Autodesk Fusion 360 part; units mm, degrees
(part 2 of 4)
sketch "Sketch7" plane through (0, 0, 2.5) normal (0, 0, 1) x (-1, 0, 0)
  line L0 (-32.4248, -53.9298) -> (-46.6248, -53.9298)
  line L1 (-46.6248, -53.9298) -> (-46.6248, -39.7298)
  line L2 (-46.6248, -39.7298) -> (-32.4248, -39.7298)
  line L3 (-32.4248, -39.7298) -> (-32.4248, -53.9298)
  line L4 (5.5752, -42.9298) -> (-8.6248, -42.9298)
  line L5 (-8.6248, -42.9298) -> (-8.6248, -28.7298)
  line L6 (-8.6248, -28.7298) -> (5.5752, -28.7298)
  line L7 (5.5752, -28.7298) -> (5.5752, -42.9298)
  line L8 (-32.4248, -15.9298) -> (-46.6248, -15.9298)
  line L9 (-46.6248, -15.9298) -> (-46.6248, -1.7298)
  line L10 (-46.6248, -1.7298) -> (-32.4248, -1.7298)
  line L11 (-32.4248, -1.7298) -> (-32.4248, -15.9298)
  line L12 (43.5752, 5.0702) -> (29.3752, 5.0702)
  line L13 (29.3752, 5.0702) -> (29.3752, 19.2702)
  line L14 (29.3752, 19.2702) -> (43.5752, 19.2702)
  line L15 (43.5752, 19.2702) -> (43.5752, 5.0702)
  line L16 (69.4872, 20.2441) -> (57.0872, 20.2441)
  line L17 (57.0872, 20.2441) -> (57.0872, 32.3441)
  line L18 (57.0872, 32.3441) -> (69.4872, 32.3441)
  line L19 (69.4872, 32.3441) -> (69.4872, 20.2441)
  line L20 (-13.4248, -57.9298) -> (-27.6248, -57.9298)
  line L21 (-27.6248, -57.9298) -> (-27.6248, -43.7298)
  line L22 (-27.6248, -43.7298) -> (-13.4248, -43.7298)
  line L23 (-13.4248, -43.7298) -> (-13.4248, -57.9298)
  line L24 (-51.4248, -15.9298) -> (-65.6248, -15.9298)
  line L25 (-65.6248, -15.9298) -> (-65.6248, -1.7298)
  line L26 (-65.6248, -1.7298) -> (-51.4248, -1.7298)
  line L27 (-51.4248, -1.7298) -> (-51.4248, -15.9298)
  line L28 (-13.4248, -38.9298) -> (-27.6248, -38.9298)
  line L29 (-27.6248, -38.9298) -> (-27.6248, -24.7298)
  line L30 (-27.6248, -24.7298) -> (-13.4248, -24.7298)
  line L31 (-13.4248, -24.7298) -> (-13.4248, -38.9298)
  line L32 (43.5752, -51.9298) -> (29.3752, -51.9298)
  line L33 (29.3752, -51.9298) -> (29.3752, -37.7298)
  line L34 (29.3752, -37.7298) -> (43.5752, -37.7298)
  line L35 (43.5752, -37.7298) -> (43.5752, -51.9298)
  line L36 (5.5752, -4.9298) -> (-8.6248, -4.9298)
  line L37 (-8.6248, -4.9298) -> (-8.6248, 9.2702)
  line L38 (-8.6248, 9.2702) -> (5.5752, 9.2702)
  line L39 (5.5752, 9.2702) -> (5.5752, -4.9298)
  line L40 (24.5752, -16.9298) -> (10.3752, -16.9298)
  line L41 (10.3752, -16.9298) -> (10.3752, -2.7298)
  line L42 (10.3752, -2.7298) -> (24.5752, -2.7298)
  line L43 (24.5752, -2.7298) -> (24.5752, -16.9298)
  line L44 (-13.4248, -19.9298) -> (-27.6248, -19.9298)
  line L45 (-27.6248, -19.9298) -> (-27.6248, -5.7298)
  line L46 (-27.6248, -5.7298) -> (-13.4248, -5.7298)
  line L47 (-13.4248, -5.7298) -> (-13.4248, -19.9298)
  line L48 (5.5752, -61.9298) -> (-8.6248, -61.9298)
  line L49 (-8.6248, -61.9298) -> (-8.6248, -47.7298)
  line L50 (-8.6248, -47.7298) -> (5.5752, -47.7298)
  line L51 (5.5752, -47.7298) -> (5.5752, -61.9298)
  line L52 (-13.4248, -0.9298) -> (-27.6248, -0.9298)
  line L53 (-27.6248, -0.9298) -> (-27.6248, 13.2702)
  line L54 (-27.6248, 13.2702) -> (-13.4248, 13.2702)
  line L55 (-13.4248, 13.2702) -> (-13.4248, -0.9298)
  line L56 (24.5752, -35.9298) -> (10.3752, -35.9298)
  line L57 (10.3752, -35.9298) -> (10.3752, -21.7298)
  line L58 (10.3752, -21.7298) -> (24.5752, -21.7298)
  line L59 (24.5752, -21.7298) -> (24.5752, -35.9298)
  line L60 (-51.4248, 3.0702) -> (-65.6248, 3.0702)
  line L61 (-65.6248, 3.0702) -> (-65.6248, 17.2702)
  line L62 (-65.6248, 17.2702) -> (-51.4248, 17.2702)
  line L63 (-51.4248, 17.2702) -> (-51.4248, 3.0702)
  line L64 (50.9803, 40.3514) -> (38.6784, 33.259)
  line L65 (38.6784, 33.259) -> (31.586, 45.5609)
  line L66 (31.586, 45.5609) -> (43.8879, 52.6533)
  line L67 (43.8879, 52.6533) -> (50.9803, 40.3514)
  line L68 (34.52, 30.8616) -> (22.218, 23.7692)
  line L69 (22.218, 23.7692) -> (15.1256, 36.0711)
  line L70 (15.1256, 36.0711) -> (27.4276, 43.1635)
  line L71 (27.4276, 43.1635) -> (34.52, 30.8616)
  line L72 (-51.4248, -34.9298) -> (-65.6248, -34.9298)
  line L73 (-65.6248, -34.9298) -> (-65.6248, -20.7298)
  line L74 (-65.6248, -20.7298) -> (-51.4248, -20.7298)
  line L75 (-51.4248, -20.7298) -> (-51.4248, -34.9298)
  line L76 (-32.4248, -34.9298) -> (-46.6248, -34.9298)
  line L77 (-46.6248, -34.9298) -> (-46.6248, -20.7298)
  line L78 (-46.6248, -20.7298) -> (-32.4248, -20.7298)
  line L79 (-32.4248, -20.7298) -> (-32.4248, -34.9298)
  line L80 (43.5752, -32.9298) -> (29.3752, -32.9298)
  line L81 (29.3752, -32.9298) -> (29.3752, -18.7298)
  line L82 (29.3752, -18.7298) -> (43.5752, -18.7298)
  line L83 (43.5752, -18.7298) -> (43.5752, -32.9298)
  line L84 (5.5752, -23.9298) -> (-8.6248, -23.9298)
  line L85 (-8.6248, -23.9298) -> (-8.6248, -9.7298)
  line L86 (-8.6248, -9.7298) -> (5.5752, -9.7298)
  line L87 (5.5752, -9.7298) -> (5.5752, -23.9298)
  line L88 (-32.4248, 3.0702) -> (-46.6248, 3.0702)
  line L89 (-46.6248, 3.0702) -> (-46.6248, 17.2702)
  line L90 (-46.6248, 17.2702) -> (-32.4248, 17.2702)
  line L91 (-32.4248, 17.2702) -> (-32.4248, 3.0702)
  line L92 (66.2388, 51.9258) -> (53.9369, 44.8334)
  line L93 (53.9369, 44.8334) -> (46.8445, 57.1354)
  line L94 (46.8445, 57.1354) -> (59.1465, 64.2278)
  line L95 (59.1465, 64.2278) -> (66.2388, 51.9258)
  line L96 (24.5752, 2.0702) -> (10.3752, 2.0702)
  line L97 (10.3752, 2.0702) -> (10.3752, 16.2702)
  line L98 (10.3752, 16.2702) -> (24.5752, 16.2702)
  line L99 (24.5752, 16.2702) -> (24.5752, 2.0702)
  line L100 (43.5752, -13.9298) -> (29.3752, -13.9298)
  line L101 (29.3752, -13.9298) -> (29.3752, 0.2702)
  line L102 (29.3752, 0.2702) -> (43.5752, 0.2702)
  line L103 (43.5752, 0.2702) -> (43.5752, -13.9298)
  line L104 (-51.4248, -53.9298) -> (-65.6248, -53.9298)
  line L105 (-65.6248, -53.9298) -> (-65.6248, -39.7298)
  line L106 (-65.6248, -39.7298) -> (-51.4248, -39.7298)
  line L107 (-51.4248, -39.7298) -> (-51.4248, -53.9298)
  line L108 (24.5752, -54.9298) -> (10.3752, -54.9298)
  line L109 (10.3752, -54.9298) -> (10.3752, -40.7298)
  line L110 (10.3752, -40.7298) -> (24.5752, -40.7298)
  line L111 (24.5752, -40.7298) -> (24.5752, -54.9298)
  line L112 (42.3648, 60.1005) -> (44.7684, 55.9312)
  line L113 (44.7684, 55.9312) -> (11.8477, 36.9516)
  line L114 (11.8477, 36.9516) -> (11.8477, 20.906)
  line L115 (11.8477, 20.906) -> (2.7791, 15.6702)
  line L116 (2.7791, 15.6702) -> (-30.0248, 15.6702)
  line L117 (-30.0248, 15.6702) -> (-30.0248, 19.6702)
  line L118 (-30.0248, 19.6702) -> (-68.0248, 19.6702)
  line L119 (-68.0248, 19.6702) -> (-68.0248, -70.3298)
  line L120 (-68.0248, -70.3298) -> (7.9752, -70.3298)
  line L121 (7.9752, -70.3298) -> (7.9752, -57.3298)
  line L122 (7.9752, -57.3298) -> (26.9752, -57.3298)
  line L123 (26.9752, -57.3298) -> (26.9752, -54.3298)
  line L124 (26.9752, -54.3298) -> (45.9752, -54.3298)
  line L125 (45.9752, -54.3298) -> (45.9752, 1.8653)
  line L126 (45.9752, 1.8653) -> (75.7872, 19.0772)
  line L127 (75.7872, 19.0772) -> (75.7872, 40.1691)
  line L128 (75.7872, 40.1691) -> (58.8251, 69.5903)
  line L129 (58.8251, 69.5903) -> (42.3648, 60.1005)
  line L130 (77.7872, 17.9225) -> (77.7872, 40.7043)
  line L131 (77.7872, 40.7043) -> (59.5589, 72.3219)
  line L132 (59.5589, 72.3219) -> (39.6332, 60.8342)
  line L133 (39.6332, 60.8342) -> (42.0368, 56.665)
  line L134 (42.0368, 56.665) -> (9.8477, 38.1072)
  line L135 (9.8477, 38.1072) -> (9.8477, 22.0607)
  line L136 (9.8477, 22.0607) -> (2.2432, 17.6702)
  line L137 (2.2432, 17.6702) -> (-28.0248, 17.6702)
  line L138 (-28.0248, 17.6702) -> (-28.0248, 21.6702)
  line L139 (-28.0248, 21.6702) -> (-70.0248, 21.6702)
  line L140 (-70.0248, 21.6702) -> (-70.0248, -72.3298)
  line L141 (-70.0248, -72.3298) -> (9.9752, -72.3298)
  line L142 (9.9752, -72.3298) -> (9.9752, -59.3298)
  line L143 (9.9752, -59.3298) -> (28.9752, -59.3298)
  line L144 (28.9752, -59.3298) -> (28.9752, -56.3298)
  line L145 (28.9752, -56.3298) -> (47.9752, -56.3298)
  line L146 (47.9752, -56.3298) -> (47.9752, 0.7106)
  line L147 (47.9752, 0.7106) -> (77.7872, 17.9225)
  line L148 (39.6332, 60.8342) -> (34.4351, 57.8374)
  line L149 (34.4351, 57.8374) -> (36.8388, 53.6682)
  line L150 (39.5704, 52.9345) -> (36.1678, 58.8364)
  line L151 (42.3648, 60.1005) -> (35.4341, 56.1048)
  line L152 (-28.0248, 21.6702) -> (-24.0248, 21.6702)
  line L153 (-24.0248, 21.6702) -> (-24.0248, 17.6702)
  line L154 (-26.0248, 15.6702) -> (-26.0248, 19.6702)
  line L155 (-26.0248, 19.6702) -> (-30.0248, 19.6702)
  line L156 (28.9752, -59.3298) -> (28.9752, -64.3298)
  line L157 (28.9752, -64.3298) -> (9.9752, -64.3298)
  line L158 (26.9752, -57.3298) -> (26.9752, -62.3298)
  line L159 (26.9752, -62.3298) -> (7.9752, -62.3298)
  dimension "d122" = 2
  dimension "d197" = 6
  dimension "d198" = 2
  dimension "d199" = 2
  dimension "d200" = 4
  dimension "d201" = 2
  dimension "d202" = 8
  dimension "d203" = 8
  constraint perpendicular L133 L148
  constraint coincident L134 L149.end
  constraint perpendicular L134 L149
  constraint coincident L113 L150.start
  constraint coincident L148 L150.end
  constraint perpendicular L148 L150
  constraint coincident L112.start L129.end
  constraint coincident L149 L151.end
  constraint perpendicular L149 L151
  constraint perpendicular L138 L152
  constraint coincident L137 L153.end
  constraint perpendicular L137 L153
  constraint coincident L116 L154.start
  constraint perpendicular L116 L154
  constraint coincident L117.end L118.start
  constraint perpendicular L117 L155
  constraint perpendicular L143 L156
  constraint coincident L142 L157.end
  constraint perpendicular L142 L157
  constraint coincident L122.end L123.start
  constraint perpendicular L122 L158
  constraint coincident L121 L159.end
  constraint perpendicular L121 L159
  measures "d197" distance of L133 L149
  measures "d198" distance of L149 L150
  measures "d199" distance of L153 L154
  measures "d200" distance of L154.end L117.end
  measures "d201" distance of L157 L159
  measures "d202" distance of L145 L157
  measures "d203" distance of L141 L157
extrude "Extrude6" add sketch "Sketch7" against normal blind 2.5 contours L123 L124 L125 L126 L127 L128 L129 L130 L131 L132 L133 L143 L144 L145 L146 L147 L151 L158 | L112 L113 L133 L134 L150 L151 | L133 L148 L150 L151 | L133 L134 L150 L151 | L113 L114 L115 L116 L134 L135 L136 L137 L150 L154 | L148 L149 L150 L151 | L134 L149 L150 L151 | L116 L117 L137 L138 L154 L155 | L137 L138 L152 L153 L154 L155 | L137 L138 L154 L155 | L121 L122 L142 L143 L158 L159 | L118 L119 L120 L121 L138 L139 L140 L141 L142 L155 L159 | L142 L143 L158 L159 | L142 L143 L156 L157 L158 L159 bodies 1
sketch "Sketch8" plane through (0, 0, 0) normal (0, 0, -1) x (1, 0, 0)
  line L0 (-77.7872, 17.9225) -> (-47.9752, 0.7106)
  line L1 (-47.9752, 0.7106) -> (-47.9752, -56.3298)
  line L2 (-47.9752, -56.3298) -> (-28.9752, -56.3298)
  line L3 (-28.9752, -56.3298) -> (-28.9752, -64.3298)
  line L4 (-9.9752, -64.3298) -> (-9.9752, -72.3298)
  line L5 (-9.9752, -72.3298) -> (70.0248, -72.3298)
  line L6 (70.0248, -72.3298) -> (70.0248, 21.6702)
  line L7 (70.0248, 21.6702) -> (24.0248, 21.6702)
  line L8 (24.0248, 17.6702) -> (-2.2432, 17.6702)
  line L9 (-2.2432, 17.6702) -> (-9.8477, 22.0607)
  line L10 (-9.8477, 22.0607) -> (-9.8477, 38.1072)
  line L11 (-9.8477, 38.1072) -> (-36.8388, 53.6682)
  line L12 (-34.4351, 57.8374) -> (-59.5589, 72.3219)
  line L13 (-59.5589, 72.3219) -> (-77.7872, 40.7043)
  line L14 (-77.7872, 40.7043) -> (-77.7872, 17.9225)
  line L15 (-55.0372, 33.2941) -> (-55.0372, 19.2941)
  line L16 (-55.0372, 19.2941) -> (-71.0372, 19.2941)
  line L17 (-71.0372, 19.2941) -> (-71.0372, 33.2941)
  line L18 (-71.0372, 33.2941) -> (-55.0372, 33.2941)
  line L19 (-25.0752, -40.2298) -> (-9.8752, -40.2298)
  line L20 (-9.8752, -40.2298) -> (-9.8752, -55.4298)
  line L21 (-9.8752, -55.4298) -> (-25.0752, -55.4298)
  line L22 (-25.0752, -55.4298) -> (-25.0752, -40.2298)
  line L23 (-6.0752, -47.2298) -> (9.1248, -47.2298)
  line L24 (9.1248, -47.2298) -> (9.1248, -62.4298)
  line L25 (9.1248, -62.4298) -> (-6.0752, -62.4298)
  line L26 (-6.0752, -62.4298) -> (-6.0752, -47.2298)
  line L27 (31.9248, -20.2298) -> (47.1248, -20.2298)
  line L28 (47.1248, -20.2298) -> (47.1248, -35.4298)
  line L29 (47.1248, -35.4298) -> (31.9248, -35.4298)
  line L30 (31.9248, -35.4298) -> (31.9248, -20.2298)
  line L31 (50.9248, 2.5702) -> (50.9248, 17.7702)
  line L32 (50.9248, 17.7702) -> (66.1248, 17.7702)
  line L33 (66.1248, 17.7702) -> (66.1248, 2.5702)
  line L34 (66.1248, 2.5702) -> (50.9248, 2.5702)
  line L35 (12.9248, 13.7702) -> (28.1248, 13.7702)
  line L36 (28.1248, 13.7702) -> (28.1248, -1.4298)
  line L37 (28.1248, -1.4298) -> (12.9248, -1.4298)
  line L38 (12.9248, -1.4298) -> (12.9248, 13.7702)
  line L39 (-25.0752, 16.7702) -> (-9.8752, 16.7702)
  line L40 (-9.8752, 16.7702) -> (-9.8752, 1.5702)
  line L41 (-9.8752, 1.5702) -> (-25.0752, 1.5702)
  line L42 (-25.0752, 1.5702) -> (-25.0752, 16.7702)
  line L43 (-59.3299, 64.9107) -> (-46.1616, 57.3188)
  line L44 (-46.1616, 57.3188) -> (-53.7535, 44.1505)
  line L45 (-53.7535, 44.1505) -> (-66.9217, 51.7424)
  line L46 (-66.9217, 51.7424) -> (-59.3299, 64.9107)
  line L47 (-44.0752, 19.7702) -> (-28.8752, 19.7702)
  line L48 (-28.8752, 19.7702) -> (-28.8752, 4.5702)
  line L49 (-28.8752, 4.5702) -> (-44.0752, 4.5702)
  line L50 (-44.0752, 4.5702) -> (-44.0752, 19.7702)
  line L51 (-6.0752, 9.7702) -> (9.1248, 9.7702)
  line L52 (9.1248, 9.7702) -> (9.1248, -5.4298)
  line L53 (9.1248, -5.4298) -> (-6.0752, -5.4298)
  line L54 (-6.0752, -5.4298) -> (-6.0752, 9.7702)
  line L55 (31.9248, 2.5702) -> (31.9248, 17.7702)
  line L56 (31.9248, 17.7702) -> (47.1248, 17.7702)
  line L57 (47.1248, 17.7702) -> (47.1248, 2.5702)
  line L58 (47.1248, 2.5702) -> (31.9248, 2.5702)
  line L59 (50.9248, -20.2298) -> (66.1248, -20.2298)
  line L60 (66.1248, -20.2298) -> (66.1248, -35.4298)
  line L61 (66.1248, -35.4298) -> (50.9248, -35.4298)
  line L62 (50.9248, -35.4298) -> (50.9248, -20.2298)
  line L63 (-6.0752, -28.2298) -> (9.1248, -28.2298)
  line L64 (9.1248, -28.2298) -> (9.1248, -43.4298)
  line L65 (9.1248, -43.4298) -> (-6.0752, -43.4298)
  line L66 (-6.0752, -43.4298) -> (-6.0752, -28.2298)
  line L67 (-44.0752, -37.2298) -> (-28.8752, -37.2298)
  line L68 (-28.8752, -37.2298) -> (-28.8752, -52.4298)
  line L69 (-28.8752, -52.4298) -> (-44.0752, -52.4298)
  line L70 (-44.0752, -52.4298) -> (-44.0752, -37.2298)
  line L71 (-25.0752, -21.2298) -> (-9.8752, -21.2298)
  line L72 (-9.8752, -21.2298) -> (-9.8752, -36.4298)
  line L73 (-9.8752, -36.4298) -> (-25.0752, -36.4298)
  line L74 (-25.0752, -36.4298) -> (-25.0752, -21.2298)
  line L75 (12.9248, -24.2298) -> (28.1248, -24.2298)
  line L76 (28.1248, -24.2298) -> (28.1248, -39.4298)
  line L77 (28.1248, -39.4298) -> (12.9248, -39.4298)
  line L78 (12.9248, -39.4298) -> (12.9248, -24.2298)
  line L79 (31.9248, -39.2298) -> (47.1248, -39.2298)
  line L80 (47.1248, -39.2298) -> (47.1248, -54.4298)
  line L81 (47.1248, -54.4298) -> (31.9248, -54.4298)
  line L82 (31.9248, -54.4298) -> (31.9248, -39.2298)
  line L83 (50.9248, -1.2298) -> (66.1248, -1.2298)
  line L84 (66.1248, -1.2298) -> (66.1248, -16.4298)
  line L85 (66.1248, -16.4298) -> (50.9248, -16.4298)
  line L86 (50.9248, -16.4298) -> (50.9248, -1.2298)
  line L87 (-6.0752, -9.2298) -> (9.1248, -9.2298)
  line L88 (9.1248, -9.2298) -> (9.1248, -24.4298)
  line L89 (9.1248, -24.4298) -> (-6.0752, -24.4298)
  line L90 (-6.0752, -24.4298) -> (-6.0752, -9.2298)
  line L91 (-44.0752, -14.4298) -> (-44.0752, 0.7702)
  line L92 (-44.0752, 0.7702) -> (-28.8752, 0.7702)
  line L93 (-28.8752, 0.7702) -> (-28.8752, -14.4298)
  line L94 (-28.8752, -14.4298) -> (-44.0752, -14.4298)
  line L95 (-38.4949, 32.5761) -> (-51.6632, 40.1679)
  line L96 (-51.6632, 40.1679) -> (-44.0714, 53.3362)
  line L97 (-44.0714, 53.3362) -> (-30.9031, 45.7444)
  line L98 (-30.9031, 45.7444) -> (-38.4949, 32.5761)
  line L99 (-27.611, 43.8464) -> (-14.4427, 36.2546)
  line L100 (-14.4427, 36.2546) -> (-22.0346, 23.0863)
  line L101 (-22.0346, 23.0863) -> (-35.2029, 30.6781)
  line L102 (-35.2029, 30.6781) -> (-27.611, 43.8464)
  line L103 (-25.0752, -2.2298) -> (-9.8752, -2.2298)
  line L104 (-9.8752, -2.2298) -> (-9.8752, -17.4298)
  line L105 (-9.8752, -17.4298) -> (-25.0752, -17.4298)
  line L106 (-25.0752, -17.4298) -> (-25.0752, -2.2298)
  line L107 (12.9248, -5.2298) -> (28.1248, -5.2298)
  line L108 (28.1248, -5.2298) -> (28.1248, -20.4298)
  line L109 (28.1248, -20.4298) -> (12.9248, -20.4298)
  line L110 (12.9248, -20.4298) -> (12.9248, -5.2298)
  line L111 (31.9248, -1.2298) -> (47.1248, -1.2298)
  line L112 (47.1248, -1.2298) -> (47.1248, -16.4298)
  line L113 (47.1248, -16.4298) -> (31.9248, -16.4298)
  line L114 (31.9248, -16.4298) -> (31.9248, -1.2298)
  line L115 (50.9248, -39.2298) -> (66.1248, -39.2298)
  line L116 (66.1248, -39.2298) -> (66.1248, -54.4298)
  line L117 (66.1248, -54.4298) -> (50.9248, -54.4298)
  line L118 (50.9248, -54.4298) -> (50.9248, -39.2298)
  line L119 (12.9248, -43.2298) -> (28.1248, -43.2298)
  line L120 (28.1248, -43.2298) -> (28.1248, -58.4298)
  line L121 (28.1248, -58.4298) -> (12.9248, -58.4298)
  line L122 (12.9248, -58.4298) -> (12.9248, -43.2298)
  line L123 (-44.0752, -18.2298) -> (-28.8752, -18.2298)
  line L124 (-28.8752, -18.2298) -> (-28.8752, -33.4298)
  line L125 (-28.8752, -33.4298) -> (-44.0752, -33.4298)
  line L126 (-44.0752, -33.4298) -> (-44.0752, -18.2298)
  line L127 (-42.0916, 60.1739) -> (-58.8985, 69.8635)
  line L128 (-58.8985, 69.8635) -> (-75.9872, 40.2226)
  line L129 (-75.9872, 40.2226) -> (-75.9872, 18.9618)
  line L130 (-75.9872, 18.9618) -> (-46.1752, 1.7498)
  line L131 (-46.1752, 1.7498) -> (-46.1752, -54.5298)
  line L132 (-46.1752, -54.5298) -> (-27.1752, -54.5298)
  line L133 (-27.1752, -54.5298) -> (-27.1752, -57.5298)
  line L134 (-27.1752, -57.5298) -> (-8.1752, -57.5298)
  line L135 (-8.1752, -57.5298) -> (-8.1752, -70.5298)
  line L136 (-8.1752, -70.5298) -> (68.2248, -70.5298)
  line L137 (68.2248, -70.5298) -> (68.2248, 19.8702)
  line L138 (68.2248, 19.8702) -> (29.8248, 19.8702)
  line L139 (29.8248, 19.8702) -> (29.8248, 15.8702)
  line L140 (29.8248, 15.8702) -> (-2.7255, 15.8702)
  line L141 (-2.7255, 15.8702) -> (-11.6477, 21.0214)
  line L142 (-11.6477, 21.0214) -> (-11.6477, 37.0672)
  line L143 (-11.6477, 37.0672) -> (-44.4953, 56.0046)
  line L144 (-44.4953, 56.0046) -> (-42.0916, 60.1739)
  line L145 (-28.9752, -64.3298) -> (-9.9752, -64.3298)
  line L146 (24.0248, 21.6702) -> (24.0248, 17.6702)
  line L147 (-36.8388, 53.6682) -> (-34.4351, 57.8374)
  line L148 (-42.0916, 60.1739) -> (-42.0916, 54.6188)
  constraint coincident L143 L148.end
  constraint vertical L148
extrude "Extrude7" add sketch "Sketch8" along normal blind 5 contours L0 L1 L2 L3 L4 L5 L6 L7 L8 L9 L10 L11 L12 L13 L14 L145 L146 L147 bodies 1
fillet "Fillet25" radius 1 18 edges at (-9.9752, 64.3298, -1.25) (-9.9752, 72.3298, -1.25) (-28.9752, 64.3298, -1.25) (-28.9752, 56.3298, -1.25) (-47.9752, 56.3298, -1.25) (-47.9752, -0.7106, -1.25) (-77.7872, -17.9225, -1.25) (-77.7872, -40.7043, -1.25) (-59.5589, -72.3219, -1.25) (-36.8388, -53.6682, -1.25) (-34.4351, -57.8374, -1.25) (-9.8477, -38.1072, -1.25) (-9.8477, -22.0607, -1.25) (-2.2432, -17.6702, -1.25) (24.0248, -17.6702, -1.25) (24.0248, -21.6702, -1.25) (70.0248, -21.6702, -1.25) (70.0248, 72.3298, -1.25) on bodies 1
fillet "Fillet26" radius 0.8 6 edges at (29.8248, -15.8702, -2.5) (-2.7255, -15.8702, -2.5) (-11.6477, -21.0214, -2.5) (-46.1752, -1.7498, -2.5) (-27.1752, 54.5298, -2.5) (-8.1752, 57.5298, -2.5) on bodies 1
fillet "Fillet30" radius 0.8 1 edges at (-42.0916, -54.6188, -2.5) on bodies 1
fillet "Fillet13" radius 1.2 9 edges at (-11.6477, -37.0672, -2.5) (-58.8985, -69.8635, -2.5) (-75.9872, -40.2226, -2.5) (-75.9872, -18.9618, -2.5) (-46.1752, 54.5298, -2.5) (-8.1752, 70.5298, -2.5) (68.2248, 70.5298, -2.5) (68.2248, -19.8702, -2.5) (29.8248, -19.8702, -2.5) on bodies 1
fillet "Fillet31" radius 1.2 1 edges at (-42.0916, -60.1739, -2.5) on bodies 1
fillet "Fillet15" radius 1 108 edges at (-43.5752, 51.9298, 1.9) (-43.5752, 37.7298, 1.9) (-29.3752, 37.7298, 1.9) (-29.3752, 51.9298, 1.9) (-24.5752, 54.9298, 1.9) (-24.5752, 40.7298, 1.9) (-10.3752, 40.7298, 1.9) (-10.3752, 54.9298, 1.9) (-5.5752, 47.7298, 1.9) (-5.5752, 61.9298, 1.9) (8.6248, 61.9298, 1.9) (8.6248, 47.7298, 1.9) (13.4248, 43.7298, 1.9) (13.4248, 57.9298, 1.9) (27.6248, 57.9298, 1.9) (27.6248, 43.7298, 1.9) (32.4248, 39.7298, 1.9) (32.4248, 53.9298, 1.9) (46.6248, 53.9298, 1.9) (46.6248, 39.7298, 1.9) (51.4248, 53.9298, 1.9) (51.4248, 39.7298, 1.9) (65.6248, 39.7298, 1.9) (65.6248, 53.9298, 1.9) (65.6248, 34.9298, 1.9) (51.4248, 34.9298, 1.9) (51.4248, 20.7298, 1.9) (65.6248, 20.7298, 1.9) (46.6248, 34.9298, 1.9) (32.4248, 34.9298, 1.9) (32.4248, 20.7298, 1.9) (46.6248, 20.7298, 1.9) (27.6248, 38.9298, 1.9) (13.4248, 38.9298, 1.9) (13.4248, 24.7298, 1.9) (27.6248, 24.7298, 1.9) (8.6248, 42.9298, 1.9) (8.6248, 28.7298, 1.9) (-5.5752, 28.7298, 1.9) (-5.5752, 42.9298, 1.9) (-10.3752, 35.9298, 1.9) (-24.5752, 35.9298, 1.9) (-24.5752, 21.7298, 1.9) (-10.3752, 21.7298, 1.9) (-43.5752, 18.7298, 1.9) (-43.5752, 32.9298, 1.9) (-29.3752, 32.9298, 1.9) (-29.3752, 18.7298, 1.9) (-43.5752, 13.9298, 1.9) (-43.5752, -0.2702, 1.9) (-29.3752, -0.2702, 1.9) (-29.3752, 13.9298, 1.9) (-24.5752, 16.9298, 1.9) (-24.5752, 2.7298, 1.9) (-10.3752, 2.7298, 1.9) (-10.3752, 16.9298, 1.9) (-5.5752, 9.7298, 1.9) (-5.5752, 23.9298, 1.9) (8.6248, 23.9298, 1.9) (8.6248, 9.7298, 1.9) (13.4248, 19.9298, 1.9) (13.4248, 5.7298, 1.9) (27.6248, 5.7298, 1.9) (32.4248, 1.7298, 1.9) (27.6248, 19.9298, 1.9) (32.4248, 15.9298, 1.9) (46.6248, 15.9298, 1.9) (46.6248, 1.7298, 1.9) (51.4248, 1.7298, 1.9) (51.4248, 15.9298, 1.9) (65.6248, 15.9298, 1.9) (65.6248, 1.7298, 1.9) (65.6248, -3.0702, 1.9) (65.6248, -17.2702, 1.9) (51.4248, -3.0702, 1.9) (46.6248, -3.0702, 1.9) (51.4248, -17.2702, 1.9) (46.6248, -17.2702, 1.9) (32.4248, -3.0702, 1.9) (32.4248, -17.2702, 1.9) (27.6248, -13.2702, 1.9) (27.6248, 0.9298, 1.9) (13.4248, 0.9298, 1.9) (13.4248, -13.2702, 1.9) (8.6248, -9.2702, 1.9) (8.6248, 4.9298, 1.9) (-5.5752, 4.9298, 1.9) (-5.5752, -9.2702, 1.9) (-10.3752, -2.0702, 1.9) (-10.3752, -16.2702, 1.9) (-24.5752, -2.0702, 1.9) (-24.5752, -16.2702, 1.9) (-29.3752, -5.0702, 1.9) (-43.5752, -5.0702, 1.9) (-43.5752, -19.2702, 1.9) (-29.3752, -19.2702, 1.9) (-22.218, -23.7692, 1.9) (-15.1256, -36.0711, 1.9) (-27.4276, -43.1635, 1.9) (-34.52, -30.8616, 1.9) (-38.6784, -33.259, 1.9) (-31.586, -45.5609, 1.9) (-43.8879, -52.6533, 1.9) (-50.9803, -40.3514, 1.9) (-53.9369, -44.8334, 1.9) (-46.8445, -57.1354, 1.9) (-59.1465, -64.2278, 1.9) (-66.2388, -51.9258, 1.9) on bodies 1
fillet "Fillet16" radius 1 4 edges at (-57.0872, -20.2441, 2) (-69.4872, -20.2441, 2) (-69.4872, -32.3441, 2) (-57.0872, -32.3441, 2) on bodies 1
sketch "Sketch9" plane through (0, 0, 2.5) normal (0, 0, 1) x (-1, 0, 0)
  line L0 (-14.4248, -38.9298) -> (-26.6248, -38.9298)
  arc A0 (-27.6248, -37.9298) -> (-26.6248, -38.9298) centre (-26.6248, -37.9298) ccw
  line L1 (-27.6248, -37.9298) -> (-27.6248, -25.7298)
  arc A1 (-26.6248, -24.7298) -> (-27.6248, -25.7298) centre (-26.6248, -25.7298) ccw
  line L2 (-26.6248, -24.7298) -> (-14.4248, -24.7298)
  arc A2 (-13.4248, -25.7298) -> (-14.4248, -24.7298) centre (-14.4248, -25.7298) ccw
  line L3 (-13.4248, -25.7298) -> (-13.4248, -37.9298)
  arc A3 (-14.4248, -38.9298) -> (-13.4248, -37.9298) centre (-14.4248, -37.9298) ccw
  line L4 (-52.4248, 3.0702) -> (-64.6248, 3.0702)
  arc A4 (-65.6248, 4.0702) -> (-64.6248, 3.0702) centre (-64.6248, 4.0702) ccw
  line L5 (-65.6248, 4.0702) -> (-65.6248, 16.2702)
  arc A5 (-64.6248, 17.2702) -> (-65.6248, 16.2702) centre (-64.6248, 16.2702) ccw
  line L6 (-64.6248, 17.2702) -> (-52.4248, 17.2702)
  arc A6 (-51.4248, 16.2702) -> (-52.4248, 17.2702) centre (-52.4248, 16.2702) ccw
  line L7 (-51.4248, 16.2702) -> (-51.4248, 4.0702)
  arc A7 (-52.4248, 3.0702) -> (-51.4248, 4.0702) centre (-52.4248, 4.0702) ccw
  line L8 (50.114, 39.8519) -> (39.5447, 33.7585)
  arc A8 (38.1789, 34.1253) -> (39.5447, 33.7585) centre (39.0452, 34.6248) ccw
  line L9 (38.1789, 34.1253) -> (32.0854, 44.6946)
  arc A9 (32.4523, 46.0604) -> (32.0854, 44.6946) centre (32.9518, 45.1941) ccw
  line L10 (32.4523, 46.0604) -> (43.0216, 52.1539)
  arc A10 (44.3874, 51.787) -> (43.0216, 52.1539) centre (43.5211, 51.2875) ccw
  line L11 (44.3874, 51.787) -> (50.4809, 41.2177)
  arc A11 (50.114, 39.8519) -> (50.4809, 41.2177) centre (49.6145, 40.7182) ccw
  line L12 (33.6536, 30.3621) -> (23.0843, 24.2686)
  arc A12 (21.7185, 24.6355) -> (23.0843, 24.2686) centre (22.5849, 25.135) ccw
  line L13 (21.7185, 24.6355) -> (15.6251, 35.2048)
  arc A13 (15.992, 36.5706) -> (15.6251, 35.2048) centre (16.4914, 35.7043) ccw
  line L14 (15.992, 36.5706) -> (26.5612, 42.6641)
  arc A14 (27.927, 42.2972) -> (26.5612, 42.6641) centre (27.0607, 41.7977) ccw
  line L15 (27.927, 42.2972) -> (34.0205, 31.7279)
  arc A15 (33.6536, 30.3621) -> (34.0205, 31.7279) centre (33.1542, 31.2284) ccw
  line L16 (-52.4248, -34.9298) -> (-64.6248, -34.9298)
  arc A16 (-65.6248, -33.9298) -> (-64.6248, -34.9298) centre (-64.6248, -33.9298) ccw
  line L17 (-65.6248, -33.9298) -> (-65.6248, -21.7298)
  arc A17 (-64.6248, -20.7298) -> (-65.6248, -21.7298) centre (-64.6248, -21.7298) ccw
  line L18 (-64.6248, -20.7298) -> (-52.4248, -20.7298)
  arc A18 (-51.4248, -21.7298) -> (-52.4248, -20.7298) centre (-52.4248, -21.7298) ccw
  line L19 (-51.4248, -21.7298) -> (-51.4248, -33.9298)
  arc A19 (-52.4248, -34.9298) -> (-51.4248, -33.9298) centre (-52.4248, -33.9298) ccw
  line L20 (-33.4248, -34.9298) -> (-45.6248, -34.9298)
  arc A20 (-46.6248, -33.9298) -> (-45.6248, -34.9298) centre (-45.6248, -33.9298) ccw
  line L21 (-46.6248, -33.9298) -> (-46.6248, -21.7298)
  arc A21 (-45.6248, -20.7298) -> (-46.6248, -21.7298) centre (-45.6248, -21.7298) ccw
  line L22 (-45.6248, -20.7298) -> (-33.4248, -20.7298)
  arc A22 (-32.4248, -21.7298) -> (-33.4248, -20.7298) centre (-33.4248, -21.7298) ccw
  line L23 (-32.4248, -21.7298) -> (-32.4248, -33.9298)
  arc A23 (-33.4248, -34.9298) -> (-32.4248, -33.9298) centre (-33.4248, -33.9298) ccw
  line L24 (42.5752, -32.9298) -> (30.3752, -32.9298)
  arc A24 (29.3752, -31.9298) -> (30.3752, -32.9298) centre (30.3752, -31.9298) ccw
  line L25 (29.3752, -31.9298) -> (29.3752, -19.7298)
  arc A25 (30.3752, -18.7298) -> (29.3752, -19.7298) centre (30.3752, -19.7298) ccw
  line L26 (30.3752, -18.7298) -> (42.5752, -18.7298)
  arc A26 (43.5752, -19.7298) -> (42.5752, -18.7298) centre (42.5752, -19.7298) ccw
  line L27 (43.5752, -19.7298) -> (43.5752, -31.9298)
  arc A27 (42.5752, -32.9298) -> (43.5752, -31.9298) centre (42.5752, -31.9298) ccw
  line L28 (4.5752, -23.9298) -> (-7.6248, -23.9298)
  arc A28 (-8.6248, -22.9298) -> (-7.6248, -23.9298) centre (-7.6248, -22.9298) ccw
  line L29 (-8.6248, -22.9298) -> (-8.6248, -10.7298)
  arc A29 (-7.6248, -9.7298) -> (-8.6248, -10.7298) centre (-7.6248, -10.7298) ccw
  line L30 (-7.6248, -9.7298) -> (4.5752, -9.7298)
  arc A30 (5.5752, -10.7298) -> (4.5752, -9.7298) centre (4.5752, -10.7298) ccw
  line L31 (5.5752, -10.7298) -> (5.5752, -22.9298)
  arc A31 (4.5752, -23.9298) -> (5.5752, -22.9298) centre (4.5752, -22.9298) ccw
  line L32 (-33.4248, 3.0702) -> (-45.6248, 3.0702)
  arc A32 (-46.6248, 4.0702) -> (-45.6248, 3.0702) centre (-45.6248, 4.0702) ccw
  line L33 (-46.6248, 4.0702) -> (-46.6248, 16.2702)
  arc A33 (-45.6248, 17.2702) -> (-46.6248, 16.2702) centre (-45.6248, 16.2702) ccw
  line L34 (-45.6248, 17.2702) -> (-33.4248, 17.2702)
  arc A34 (-32.4248, 16.2702) -> (-33.4248, 17.2702) centre (-33.4248, 16.2702) ccw
  line L35 (-32.4248, 16.2702) -> (-32.4248, 4.0702)
  arc A35 (-33.4248, 3.0702) -> (-32.4248, 4.0702) centre (-33.4248, 4.0702) ccw
  line L36 (65.3725, 51.4263) -> (54.8032, 45.3329)
  arc A36 (53.4374, 45.6998) -> (54.8032, 45.3329) centre (54.3038, 46.1992) ccw
  line L37 (53.4374, 45.6998) -> (47.344, 56.269)
  arc A37 (47.7108, 57.6348) -> (47.344, 56.269) centre (48.2103, 56.7685) ccw
  line L38 (47.7108, 57.6348) -> (58.2801, 63.7283)
  arc A38 (59.6459, 63.3614) -> (58.2801, 63.7283) centre (58.7796, 62.862) ccw
  line L39 (59.6459, 63.3614) -> (65.7394, 52.7921)
  arc A39 (65.3725, 51.4263) -> (65.7394, 52.7921) centre (64.873, 52.2927) ccw
  line L40 (-52.4248, -53.9298) -> (-64.6248, -53.9298)
  arc A40 (-65.6248, -52.9298) -> (-64.6248, -53.9298) centre (-64.6248, -52.9298) ccw
  line L41 (-65.6248, -52.9298) -> (-65.6248, -40.7298)
  arc A41 (-64.6248, -39.7298) -> (-65.6248, -40.7298) centre (-64.6248, -40.7298) ccw
  line L42 (-64.6248, -39.7298) -> (-52.4248, -39.7298)
  arc A42 (-51.4248, -40.7298) -> (-52.4248, -39.7298) centre (-52.4248, -40.7298) ccw
  line L43 (-51.4248, -40.7298) -> (-51.4248, -52.9298)
  arc A43 (-52.4248, -53.9298) -> (-51.4248, -52.9298) centre (-52.4248, -52.9298) ccw
  line L44 (23.5752, 2.0702) -> (11.3752, 2.0702)
  arc A44 (10.3752, 3.0702) -> (11.3752, 2.0702) centre (11.3752, 3.0702) ccw
  line L45 (10.3752, 3.0702) -> (10.3752, 15.2702)
  arc A45 (11.3752, 16.2702) -> (10.3752, 15.2702) centre (11.3752, 15.2702) ccw
  line L46 (11.3752, 16.2702) -> (23.5752, 16.2702)
  arc A46 (24.5752, 15.2702) -> (23.5752, 16.2702) centre (23.5752, 15.2702) ccw
  line L47 (24.5752, 15.2702) -> (24.5752, 3.0702)
  arc A47 (23.5752, 2.0702) -> (24.5752, 3.0702) centre (23.5752, 3.0702) ccw
  line L48 (42.5752, -13.9298) -> (30.3752, -13.9298)
  arc A48 (29.3752, -12.9298) -> (30.3752, -13.9298) centre (30.3752, -12.9298) ccw
  line L49 (29.3752, -12.9298) -> (29.3752, -0.7298)
  arc A49 (30.3752, 0.2702) -> (29.3752, -0.7298) centre (30.3752, -0.7298) ccw
  line L50 (30.3752, 0.2702) -> (42.5752, 0.2702)
  arc A50 (43.5752, -0.7298) -> (42.5752, 0.2702) centre (42.5752, -0.7298) ccw
  line L51 (43.5752, -0.7298) -> (43.5752, -12.9298)
  arc A51 (42.5752, -13.9298) -> (43.5752, -12.9298) centre (42.5752, -12.9298) ccw
  line L52 (42.5752, -51.9298) -> (30.3752, -51.9298)
  arc A52 (29.3752, -50.9298) -> (30.3752, -51.9298) centre (30.3752, -50.9298) ccw
  line L53 (29.3752, -50.9298) -> (29.3752, -38.7298)
  arc A53 (30.3752, -37.7298) -> (29.3752, -38.7298) centre (30.3752, -38.7298) ccw
  line L54 (30.3752, -37.7298) -> (42.5752, -37.7298)
  arc A54 (43.5752, -38.7298) -> (42.5752, -37.7298) centre (42.5752, -38.7298) ccw
  line L55 (43.5752, -38.7298) -> (43.5752, -50.9298)
  arc A55 (42.5752, -51.9298) -> (43.5752, -50.9298) centre (42.5752, -50.9298) ccw
  line L56 (4.5752, -4.9298) -> (-7.6248, -4.9298)
  arc A56 (-8.6248, -3.9298) -> (-7.6248, -4.9298) centre (-7.6248, -3.9298) ccw
  line L57 (-8.6248, -3.9298) -> (-8.6248, 8.2702)
  arc A57 (-7.6248, 9.2702) -> (-8.6248, 8.2702) centre (-7.6248, 8.2702) ccw
  line L58 (-7.6248, 9.2702) -> (4.5752, 9.2702)
  arc A58 (5.5752, 8.2702) -> (4.5752, 9.2702) centre (4.5752, 8.2702) ccw
  line L59 (5.5752, 8.2702) -> (5.5752, -3.9298)
  arc A59 (4.5752, -4.9298) -> (5.5752, -3.9298) centre (4.5752, -3.9298) ccw
  line L60 (23.5752, -16.9298) -> (11.3752, -16.9298)
  arc A60 (10.3752, -15.9298) -> (11.3752, -16.9298) centre (11.3752, -15.9298) ccw
  line L61 (10.3752, -15.9298) -> (10.3752, -3.7298)
  arc A61 (11.3752, -2.7298) -> (10.3752, -3.7298) centre (11.3752, -3.7298) ccw
  line L62 (11.3752, -2.7298) -> (23.5752, -2.7298)
  arc A62 (24.5752, -3.7298) -> (23.5752, -2.7298) centre (23.5752, -3.7298) ccw
  line L63 (24.5752, -3.7298) -> (24.5752, -15.9298)
  arc A63 (23.5752, -16.9298) -> (24.5752, -15.9298) centre (23.5752, -15.9298) ccw
  line L64 (-14.4248, -19.9298) -> (-26.6248, -19.9298)
  arc A64 (-27.6248, -18.9298) -> (-26.6248, -19.9298) centre (-26.6248, -18.9298) ccw
  line L65 (-27.6248, -18.9298) -> (-27.6248, -6.7298)
  arc A65 (-26.6248, -5.7298) -> (-27.6248, -6.7298) centre (-26.6248, -6.7298) ccw
  line L66 (-26.6248, -5.7298) -> (-14.4248, -5.7298)
  arc A66 (-13.4248, -6.7298) -> (-14.4248, -5.7298) centre (-14.4248, -6.7298) ccw
  line L67 (-13.4248, -6.7298) -> (-13.4248, -18.9298)
  arc A67 (-14.4248, -19.9298) -> (-13.4248, -18.9298) centre (-14.4248, -18.9298) ccw
  line L68 (-14.4248, -0.9298) -> (-26.6248, -0.9298)
  arc A68 (-27.6248, 0.0702) -> (-26.6248, -0.9298) centre (-26.6248, 0.0702) ccw
  line L69 (-27.6248, 0.0702) -> (-27.6248, 12.2702)
  arc A69 (-26.6248, 13.2702) -> (-27.6248, 12.2702) centre (-26.6248, 12.2702) ccw
  line L70 (-26.6248, 13.2702) -> (-14.4248, 13.2702)
  arc A70 (-13.4248, 12.2702) -> (-14.4248, 13.2702) centre (-14.4248, 12.2702) ccw
  line L71 (-13.4248, 12.2702) -> (-13.4248, 0.0702)
  arc A71 (-14.4248, -0.9298) -> (-13.4248, 0.0702) centre (-14.4248, 0.0702) ccw
  line L72 (23.5752, -35.9298) -> (11.3752, -35.9298)
  arc A72 (10.3752, -34.9298) -> (11.3752, -35.9298) centre (11.3752, -34.9298) ccw
  line L73 (10.3752, -34.9298) -> (10.3752, -22.7298)
  arc A73 (11.3752, -21.7298) -> (10.3752, -22.7298) centre (11.3752, -22.7298) ccw
  line L74 (11.3752, -21.7298) -> (23.5752, -21.7298)
  arc A74 (24.5752, -22.7298) -> (23.5752, -21.7298) centre (23.5752, -22.7298) ccw
  line L75 (24.5752, -22.7298) -> (24.5752, -34.9298)
  arc A75 (23.5752, -35.9298) -> (24.5752, -34.9298) centre (23.5752, -34.9298) ccw
  line L76 (4.5752, -61.9298) -> (-7.6248, -61.9298)
  arc A76 (-8.6248, -60.9298) -> (-7.6248, -61.9298) centre (-7.6248, -60.9298) ccw
  line L77 (-8.6248, -60.9298) -> (-8.6248, -48.7298)
  arc A77 (-7.6248, -47.7298) -> (-8.6248, -48.7298) centre (-7.6248, -48.7298) ccw
  line L78 (-7.6248, -47.7298) -> (4.5752, -47.7298)
  arc A78 (5.5752, -48.7298) -> (4.5752, -47.7298) centre (4.5752, -48.7298) ccw
  line L79 (5.5752, -48.7298) -> (5.5752, -60.9298)
  arc A79 (4.5752, -61.9298) -> (5.5752, -60.9298) centre (4.5752, -60.9298) ccw
  line L80 (-52.4248, -15.9298) -> (-64.6248, -15.9298)
  arc A80 (-65.6248, -14.9298) -> (-64.6248, -15.9298) centre (-64.6248, -14.9298) ccw
  line L81 (-65.6248, -14.9298) -> (-65.6248, -2.7298)
  arc A81 (-64.6248, -1.7298) -> (-65.6248, -2.7298) centre (-64.6248, -2.7298) ccw
  line L82 (-64.6248, -1.7298) -> (-52.4248, -1.7298)
  arc A82 (-51.4248, -2.7298) -> (-52.4248, -1.7298) centre (-52.4248, -2.7298) ccw
  line L83 (-51.4248, -2.7298) -> (-51.4248, -14.9298)
  arc A83 (-52.4248, -15.9298) -> (-51.4248, -14.9298) centre (-52.4248, -14.9298) ccw
  line L84 (-14.4248, -57.9298) -> (-26.6248, -57.9298)
  arc A84 (-27.6248, -56.9298) -> (-26.6248, -57.9298) centre (-26.6248, -56.9298) ccw
  line L85 (-27.6248, -56.9298) -> (-27.6248, -44.7298)
  arc A85 (-26.6248, -43.7298) -> (-27.6248, -44.7298) centre (-26.6248, -44.7298) ccw
  line L86 (-26.6248, -43.7298) -> (-14.4248, -43.7298)
  arc A86 (-13.4248, -44.7298) -> (-14.4248, -43.7298) centre (-14.4248, -44.7298) ccw
  line L87 (-13.4248, -44.7298) -> (-13.4248, -56.9298)
  arc A87 (-14.4248, -57.9298) -> (-13.4248, -56.9298) centre (-14.4248, -56.9298) ccw
  line L88 (-33.4248, -15.9298) -> (-45.6248, -15.9298)
  arc A88 (-46.6248, -14.9298) -> (-45.6248, -15.9298) centre (-45.6248, -14.9298) ccw
  line L89 (-46.6248, -14.9298) -> (-46.6248, -2.7298)
  arc A89 (-45.6248, -1.7298) -> (-46.6248, -2.7298) centre (-45.6248, -2.7298) ccw
  line L90 (-45.6248, -1.7298) -> (-33.4248, -1.7298)
  arc A90 (-32.4248, -2.7298) -> (-33.4248, -1.7298) centre (-33.4248, -2.7298) ccw
  line L91 (-32.4248, -2.7298) -> (-32.4248, -14.9298)
  arc A91 (-33.4248, -15.9298) -> (-32.4248, -14.9298) centre (-33.4248, -14.9298) ccw
  line L92 (4.5752, -42.9298) -> (-7.6248, -42.9298)
  arc A92 (-8.6248, -41.9298) -> (-7.6248, -42.9298) centre (-7.6248, -41.9298) ccw
  line L93 (-8.6248, -41.9298) -> (-8.6248, -29.7298)
  arc A93 (-7.6248, -28.7298) -> (-8.6248, -29.7298) centre (-7.6248, -29.7298) ccw
  line L94 (-7.6248, -28.7298) -> (4.5752, -28.7298)
  arc A94 (5.5752, -29.7298) -> (4.5752, -28.7298) centre (4.5752, -29.7298) ccw
  line L95 (5.5752, -29.7298) -> (5.5752, -41.9298)
  arc A95 (4.5752, -42.9298) -> (5.5752, -41.9298) centre (4.5752, -41.9298) ccw
  line L96 (-33.4248, -53.9298) -> (-45.6248, -53.9298)
  arc A96 (-46.6248, -52.9298) -> (-45.6248, -53.9298) centre (-45.6248, -52.9298) ccw
  line L97 (-46.6248, -52.9298) -> (-46.6248, -40.7298)
  arc A97 (-45.6248, -39.7298) -> (-46.6248, -40.7298) centre (-45.6248, -40.7298) ccw
  line L98 (-45.6248, -39.7298) -> (-33.4248, -39.7298)
  arc A98 (-32.4248, -40.7298) -> (-33.4248, -39.7298) centre (-33.4248, -40.7298) ccw
  line L99 (-32.4248, -40.7298) -> (-32.4248, -52.9298)
  arc A99 (-33.4248, -53.9298) -> (-32.4248, -52.9298) centre (-33.4248, -52.9298) ccw
  line L100 (42.5752, 5.0702) -> (30.3752, 5.0702)
  arc A100 (29.3752, 6.0702) -> (30.3752, 5.0702) centre (30.3752, 6.0702) ccw
  line L101 (29.3752, 6.0702) -> (29.3752, 18.2702)
  arc A101 (30.3752, 19.2702) -> (29.3752, 18.2702) centre (30.3752, 18.2702) ccw
  line L102 (30.3752, 19.2702) -> (42.5752, 19.2702)
  arc A102 (43.5752, 18.2702) -> (42.5752, 19.2702) centre (42.5752, 18.2702) ccw
  line L103 (43.5752, 18.2702) -> (43.5752, 6.0702)
  arc A103 (42.5752, 5.0702) -> (43.5752, 6.0702) centre (42.5752, 6.0702) ccw
  line L104 (68.4872, 20.2441) -> (58.0872, 20.2441)
  arc A104 (57.0872, 21.2441) -> (58.0872, 20.2441) centre (58.0872, 21.2441) ccw
  line L105 (57.0872, 21.2441) -> (57.0872, 31.3441)
  arc A105 (58.0872, 32.3441) -> (57.0872, 31.3441) centre (58.0872, 31.3441) ccw
  line L106 (58.0872, 32.3441) -> (68.4872, 32.3441)
  arc A106 (69.4872, 31.3441) -> (68.4872, 32.3441) centre (68.4872, 31.3441) ccw
  line L107 (69.4872, 31.3441) -> (69.4872, 21.2441)
  arc A107 (68.4872, 20.2441) -> (69.4872, 21.2441) centre (68.4872, 21.2441) ccw
  line L108 (23.5752, -54.9298) -> (11.3752, -54.9298)
  arc A108 (10.3752, -53.9298) -> (11.3752, -54.9298) centre (11.3752, -53.9298) ccw
  line L109 (10.3752, -53.9298) -> (10.3752, -41.7298)
  arc A109 (11.3752, -40.7298) -> (10.3752, -41.7298) centre (11.3752, -41.7298) ccw
  line L110 (11.3752, -40.7298) -> (23.5752, -40.7298)
  arc A110 (24.5752, -41.7298) -> (23.5752, -40.7298) centre (23.5752, -41.7298) ccw
  line L111 (24.5752, -41.7298) -> (24.5752, -53.9298)
  arc A111 (23.5752, -54.9298) -> (24.5752, -53.9298) centre (23.5752, -53.9298) ccw
  line L112 (35.9725, 53.1687) -> (10.3482, 38.3957)
  line L113 (9.8477, 37.5294) -> (9.8477, 22.638)
  line L114 (9.3477, 21.772) -> (2.4752, 17.8042)
  line L115 (1.9752, 17.6702) -> (-23.0248, 17.6702)
  line L116 (-25.0248, 21.6702) -> (-69.0248, 21.6702)
  line L117 (-70.0248, 20.6702) -> (-70.0248, -71.3298)
  line L118 (-69.0248, -72.3298) -> (8.9752, -72.3298)
  line L119 (9.9752, -71.3298) -> (9.9752, -65.3298)
  line L120 (28.9752, -63.3298) -> (28.9752, -57.3298)
  line L121 (29.9752, -56.3298) -> (46.9752, -56.3298)
  line L122 (47.9752, -55.3298) -> (47.9752, 0.1332)
  line L123 (48.4752, 0.9993) -> (77.2872, 17.6338)
  line L124 (77.7872, 18.4999) -> (77.7872, 40.4367)
  line L125 (77.6535, 40.9362) -> (60.0583, 71.4556)
  line L126 (58.6925, 71.8224) -> (35.3015, 58.3369)
  line L127 (-49.2748, -72.3298) -> (-65.7748, -72.3298)
  line L128 (-65.7748, -72.3298) -> (-65.7748, -56.8298)
  line L129 (-65.7748, -56.8298) -> (-49.2748, -56.8298)
  line L130 (-49.2748, -56.8298) -> (-49.2748, -72.3298)
  line L131 (-31.8698, -72.3298) -> (-43.1798, -72.3298)
  line L132 (-43.1798, -72.3298) -> (-43.1798, -61.3298)
  line L133 (-43.1798, -61.3298) -> (-31.8698, -61.3298)
  line L134 (-31.8698, -61.3298) -> (-31.8698, -72.3298)
  line L135 (-13.8698, -72.3298) -> (-25.1798, -72.3298)
  line L136 (-25.1798, -72.3298) -> (-25.1798, -61.3298)
  line L137 (-25.1798, -61.3298) -> (-13.8698, -61.3298)
  line L138 (-13.8698, -61.3298) -> (-13.8698, -72.3298)
  line L139 (-19.5248, -61.3298) -> (-19.5248, -72.3298) construction
  line L140 (-37.5248, -72.3298) -> (-37.5248, -61.3298) construction
  line L141 (-57.5248, -72.3298) -> (-57.5248, -56.8298) construction
  line L142 (-65.6248, -46.8298) -> (-51.4248, -46.8298) construction
  line L143 (-49.0248, -56.3298) -> (-68.0248, -56.3298) construction
  line L144 (-68.0248, -56.3298) -> (-68.0248, -37.3298) construction
  line L145 (-68.0248, -37.3298) -> (-49.0248, -37.3298) construction
  line L146 (-49.0248, -37.3298) -> (-49.0248, -56.3298) construction
  line L147 (-49.0248, -56.3298) -> (-68.0248, -37.3298) construction
  line L148 (-68.0248, -56.3298) -> (-49.0248, -37.3298) construction
  arc A112 (-70.0248, -71.3298) -> (-69.0248, -72.3298) centre (-69.0248, -71.3298) ccw
  arc A113 (8.9752, -72.3298) -> (9.9752, -71.3298) centre (8.9752, -71.3298) ccw
  arc A114 (10.9752, -64.3298) -> (9.9752, -65.3298) centre (10.9752, -65.3298) ccw
  line L149 (10.9752, -64.3298) -> (27.9752, -64.3298)
  arc A115 (27.9752, -64.3298) -> (28.9752, -63.3298) centre (27.9752, -63.3298) ccw
  arc A116 (29.9752, -56.3298) -> (28.9752, -57.3298) centre (29.9752, -57.3298) ccw
  arc A117 (46.9752, -56.3298) -> (47.9752, -55.3298) centre (46.9752, -55.3298) ccw
  arc A118 (48.4752, 0.9993) -> (47.9752, 0.1332) centre (48.9752, 0.1332) ccw
  arc A119 (77.2872, 17.6338) -> (77.7872, 18.4999) centre (76.7872, 18.4999) ccw
  arc A120 (77.7872, 40.4367) -> (77.6535, 40.9362) centre (76.7872, 40.4367) ccw
  arc A121 (60.0583, 71.4556) -> (58.6925, 71.8224) centre (59.192, 70.9561) ccw
  arc A122 (35.3015, 58.3369) -> (34.9346, 56.9711) centre (35.8009, 57.4706) ccw
  line L150 (34.9346, 56.9711) -> (36.3394, 54.5345)
  arc A123 (35.9725, 53.1687) -> (36.3394, 54.5345) centre (35.473, 54.0351) ccw
  arc A124 (10.3482, 38.3957) -> (9.8477, 37.5294) centre (10.8477, 37.5294) ccw
  arc A125 (9.3477, 21.772) -> (9.8477, 22.638) centre (8.8477, 22.638) ccw
  arc A126 (1.9752, 17.6702) -> (2.4752, 17.8042) centre (1.9752, 18.6702) ccw
  arc A127 (-24.0248, 18.6702) -> (-23.0248, 17.6702) centre (-23.0248, 18.6702) ccw
  line L151 (-24.0248, 18.6702) -> (-24.0248, 20.6702)
  arc A128 (-24.0248, 20.6702) -> (-25.0248, 21.6702) centre (-25.0248, 20.6702) ccw
  arc A129 (-69.0248, 21.6702) -> (-70.0248, 20.6702) centre (-69.0248, 20.6702) ccw
  point P0 (-58.5248, -46.8298)
  dimension "d144" = 15.5
  dimension "d145" = 16.5
  dimension "d146" = 11.31
  dimension "d147" = 11
  dimension "d148" = 18
  dimension "d149" = 20
  dimension "d150" = 4.25
  dimension "d155" = 19
  constraint horizontal L127
  constraint vertical L128
  constraint horizontal L129
  constraint vertical L130
  constraint coincident L118 L127.start
  constraint horizontal L131
  constraint vertical L132
  constraint horizontal L133
  constraint vertical L134
  constraint coincident L118 L131.start
  constraint horizontal L135
  constraint vertical L136
  constraint horizontal L137
  constraint vertical L138
  constraint coincident L118 L135.start
  constraint equal L131 L135
  constraint equal L132 L136
  constraint midpoint L137 L139.start
  constraint midpoint L135 L139.end
  constraint midpoint L131 L140.start
  constraint midpoint L133 L140.end
  constraint midpoint L127 L141.start
  constraint midpoint L129 L141.end
  constraint midpoint L41 L142.start
  constraint midpoint L43 L142.end
  constraint horizontal L143
  constraint perpendicular L143 L144
  constraint parallel L143 L145
  constraint parallel L144 L146
  constraint coincident L147 P0
  constraint coincident L148 P0
  constraint midpoint L142 P0
  constraint equal L145 L146
  measures "d144" distance of L127 L129
  measures "d145" distance of L127.start L127.end
  measures "d146" distance of L131.start L131.end
  measures "d147" distance of L131.end L132.end
  measures "d148" distance of L139 L140
  measures "d149" distance of L140 L141
  measures "d150" distance of L117 L128
  measures "d155" distance of L143.end L144.end
extrude "Extrude8" add sketch "Sketch9" along normal blind 0.5 contours L118 L131 L132 L133 L134 | L118 L135 L136 L137 L138 bodies 1
extrude "Extrude9" add sketch "Sketch9" along normal blind 2.8 contours L118 L127 L128 L129 L130 bodies 1
sketch "Sketch10" plane through (0, 72.3298, 0) normal (0, 1, 0) x (-1, 0, 0)
  line L0 (8.9752, 2.5) -> (-13.8698, 2.5)
  line L1 (-13.8698, 2.5) -> (-13.8698, 3)
  line L2 (-13.8698, 3) -> (-25.1798, 3)
  line L3 (-25.1798, 3) -> (-25.1798, 2.5)
  line L4 (-25.1798, 2.5) -> (-31.8698, 2.5)
  line L5 (-31.8698, 2.5) -> (-31.8698, 3)
  line L6 (-31.8698, 3) -> (-43.1798, 3)
  line L7 (-43.1798, 3) -> (-43.1798, 2.5)
  line L8 (-43.1798, 2.5) -> (-49.2748, 2.5)
  line L9 (-49.2748, 2.5) -> (-49.2748, 5.3)
  line L10 (-49.2748, 5.3) -> (-65.7748, 5.3)
  line L11 (-65.7748, 5.3) -> (-65.7748, 2.5)
  line L12 (-69.0248, -5) -> (8.9752, -5)
  line L13 (-64.7748, 4.3) -> (-50.2748, 4.3)
  line L14 (-50.2748, 4.3) -> (-50.2748, -2.2)
  line L15 (-50.2748, -2.2) -> (-64.7748, -2.2)
  line L16 (-64.7748, -2.2) -> (-64.7748, 4.3)
  line L17 (-42.1798, 2) -> (-32.8698, 2)
  line L18 (-32.8698, 2) -> (-32.8698, -1.45)
  line L19 (-32.8698, -1.45) -> (-42.1798, -1.45)
  line L20 (-42.1798, -1.45) -> (-42.1798, 2)
  line L21 (-24.1798, 2) -> (-14.8698, 2)
  line L22 (-14.8698, 2) -> (-14.8698, -1.45)
  line L23 (-14.8698, -1.45) -> (-24.1798, -1.45)
  line L24 (-24.1798, -1.45) -> (-24.1798, 2)
  line L25 (-69.0248, 2.5) -> (-69.0248, -5)
  line L26 (8.9752, -5) -> (8.9752, 2.5)
  line L27 (-65.7748, 2.5) -> (-69.0248, 2.5)
  dimension "d156" = 1
  dimension "d157" = 1
  dimension "d158" = 1
  dimension "d159" = 6.5
  dimension "d160" = 1
  dimension "d161" = 1
  dimension "d162" = 1
  dimension "d163" = 1
  dimension "d164" = 1
  dimension "d165" = 1
  dimension "d166" = 3.45
  constraint horizontal L13
  constraint vertical L14
  constraint horizontal L15
  constraint vertical L16
  constraint horizontal L17
  constraint vertical L18
  constraint horizontal L19
  constraint vertical L20
  constraint horizontal L21
  constraint vertical L22
  constraint horizontal L23
  constraint vertical L24
  constraint equal L18 L24
  measures "d156" distance of L9 L14
  measures "d157" distance of L11 L16
  measures "d158" distance of L10 L13
  measures "d159" distance of L13 L15
  measures "d160" distance of L7 L20
  measures "d161" distance of L5 L18
  measures "d162" distance of L6 L17
  measures "d163" distance of L2 L21
  measures "d164" distance of L3 L24
  measures "d165" distance of L1 L22
  measures "d166" distance of L17 L19
extrude "Extrude10" cut sketch "Sketch10" against normal blind 15 contours L13 L14 L15 L16 bodies 1
extrude "Extrude11" cut sketch "Sketch10" against normal blind 9 contours L17 L18 L19 L20 | L21 L22 L23 L24 bodies 1
fillet "Fillet22" radius 1 39 edges at (2.4473, 72.3298, 2.5) (-9.6823, 72.0369, 2.5) (-9.9752, 68.3298, 2.5) (-10.2681, 64.6227, 2.5) (-19.4752, 64.3298, 2.5) (-28.6823, 64.0369, 2.5) (-28.9752, 60.3298, 2.5) (-29.2681, 56.6227, 2.5) (-38.4752, 56.3298, 2.5) (-47.6823, 56.0369, 2.5) (-47.9752, 27.5983, 2.5) (-48.1092, -0.6332, 2.5) (-62.8812, -9.3166, 2.5) (-77.6532, -17.9999, 2.5) (-77.7872, -29.4683, 2.5) (-77.7532, -40.6952, 2.5) (-68.8559, -56.1959, 2.5) (-59.4514, -71.9219, 2.5) (-46.997, -65.0797, 2.5) (-34.8352, -57.73, 2.5) (-35.637, -55.7528, 2.5) (-36.4388, -53.7757, 2.5) (-23.1604, -45.7822, 2.5) (-9.9818, -38.0297, 2.5) (-9.8477, -30.0837, 2.5) (-9.7137, -22.138, 2.5) (-5.9115, -19.7881, 2.5) (-2.2341, -17.7043, 2.5) (10.5248, -17.6702, 2.5) (23.7319, -17.9631, 2.5) (24.0248, -19.6702, 2.5) (24.3177, -21.3773, 2.5) (47.0248, -21.6702, 2.5) (69.7319, -21.3773, 2.5) (70.0248, 25.3298, 2.5) (69.7319, 72.0369, 2.5) (67.3998, 72.3298, 2.5) (46.2273, 72.3298, 2.5) (28.5248, 72.3298, 2.5) on bodies 1
fillet "Fillet17" radius 0.2 12 edges at (31.8698, 66.8298, 2.5) (37.5248, 61.3298, 2.5) (43.1798, 66.8298, 2.5) (25.1798, 66.8298, 2.5) (19.5248, 61.3298, 2.5) (13.8698, 66.8298, 2.5) (13.8698, 66.8298, 3) (19.5248, 61.3298, 3) (25.1798, 66.8298, 3) (37.5248, 61.3298, 3) (31.8698, 66.8298, 3) (43.1798, 66.8298, 3) on bodies 1
fillet "Fillet18" radius 0.5 10 edges at (49.2748, 64.0798, 2.5) (49.2748, 72.0369, 2.2071) (57.5248, 56.8298, 2.5) (57.5248, 56.8298, 5.3) (49.2748, 64.5798, 5.3) (49.2748, 56.8298, 3.9) (65.7748, 56.8298, 3.9) (65.7748, 64.0798, 2.5) (65.7748, 72.0369, 2.2071) (65.7748, 64.5798, 5.3) on bodies 1
fillet "Fillet20" radius 1 4 edges at (50.2748, 64.8298, 4.3) (64.7748, 64.8298, 4.3) (64.7748, 71.4298, -2.2) (50.2748, 71.4298, -2.2) on bodies 1
fillet "Fillet21" radius 1.4 8 edges at (42.1798, 67.8298, 2) (42.1798, 71.4298, -1.45) (32.8698, 67.8298, 2) (32.8698, 71.4298, -1.45) (24.1798, 67.8298, 2) (24.1798, 71.4298, -1.45) (14.8698, 67.8298, 2) (14.8698, 71.4298, -1.45) on bodies 1
fillet "Fillet23" radius 0.2 21 edges at (65.9377, 72.3298, 2.029) (65.7748, 72.3298, 3.709) (65.6283, 72.3298, 5.1536) (57.5248, 72.3298, 5.3) (49.4212, 72.3298, 5.1536) (49.2748, 72.3298, 3.709) (49.1118, 72.3298, 2.029) (43.246, 72.3298, 1.8244) (43.1798, 72.3298, 2.4817) (43.1212, 72.3298, 2.9414) (37.5248, 72.3298, 3) (31.9283, 72.3298, 2.9414) (31.8698, 72.3298, 2.4817) (31.8036, 72.3298, 1.8244) (25.2461, 72.3298, 1.8242) (25.1798, 72.3298, 2.4817) (25.1212, 72.3298, 2.9414) (19.5248, 72.3298, 3) (13.9283, 72.3298, 2.9414) (13.8698, 72.3298, 2.4817) (13.8036, 72.3298, 1.8244) on bodies 1